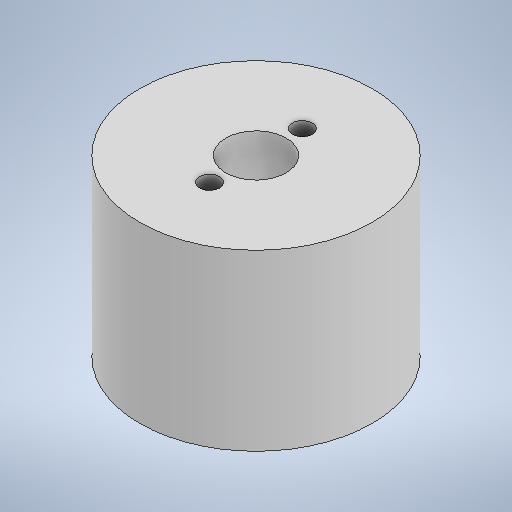
# Autodesk Inventor part: 45DegreeMirrorPost_0p75in
Saved by Autodesk Inventor 2025.2 (Build 292293000, 293)
## iProperties
Created: 2024-01-08
Part Number: 45DegreeMirrorPost_0p75in
Material: Generic
Document SubType Name: Modeling
Designer: monolithic
Density: 1 g/cm^3
Appearance: Default
Author: monolithic
Autodesk Inventor part; units mm, degrees
ref_plane "YZ Plane" through (0, 0, 0) normal (1, 0, 0) x (0, 1, 0)
ref_plane "XZ Plane" through (0, 0, 0) normal (0, 1, 0) x (-1, 0, 0)
ref_plane "XY Plane" through (0, 0, 0) normal (0, 0, 1) x (1, 0, 0)
sketch "Sketch1" plane through (0, 0, 0) normal (0, 1, 0) x (-1, 0, 0)
  circle A0 centre (0, 0) radius 12.7
  circle A1 centre (0, 0) radius 3.302
  dimension "d0" = 25.4
  dimension "d1" = 6.604
  constraints: 2 centre point, 2 coincident
  measures "d0" diameter of A0
  measures "d1" diameter of A1
extrude "Extrusion1" add sketch "Sketch1" along normal blind 19.05
sketch "Sketch2" plane through (0, 19.05, 0) normal (0, 1, 0) x (1, 0, 0)
  line L0 (0, 0) -> (0, -5.08)
  line L1 (0, -5.08) -> (0, 0)
  line L2 (0, 0) -> (0, 5.08)
  circle A0 centre (0, -5.08) radius 1.0922
  circle A1 centre (0, 5.08) radius 1.0922
  dimension "d4" = 5.08
  dimension "d5" = 5.08
  dimension "d6" = 2.1844
  dimension "d7" = 2.1844
  constraints: 6 end point, 2 centre point, 2 coincident, 1 collinear, 1 point on line, 1 vertical
  measures "d4" distance of L0.start L0.end
  measures "d5" distance of L0.start L2.end
  measures "d6" diameter of A0
  measures "d7" diameter of A1
extrude "Extrusion2" cut sketch "Sketch2" against normal blind 4.445
sketch "Sketch3" plane through (0, 0, 0) normal (0, -1, 0) x (1, 0, 0)
  line L0 (0, 0) -> (0, 5.08)
  line L1 (0, 5.08) -> (0, -5.08)
  circle A0 centre (0, 5.08) radius 1.0922
  circle A1 centre (0, -5.08) radius 1.0922
  dimension "d10" = 5.08
  dimension "d11" = 10.16
  dimension "d14" = 2.1844
  dimension "d15" = 2.1844
  constraints: 4 end point, 2 centre point, 2 coincident, 1 point on line, 1 vertical
  measures "d10" distance of L0.start L0.end
  measures "d11" distance of L0.end L1.end
  measures "d14" diameter of A1
  measures "d15" diameter of A0
extrude "Extrusion3" cut sketch "Sketch3" against normal blind 1.905
body "Solid1"
